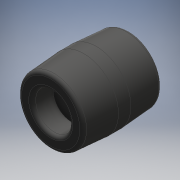
# Autodesk Inventor part: Pied
Saved by Autodesk Inventor 2016 SP1 (Build 200210100, 210)
## iProperties
Created: 2018-06-13
Part Number: Pied
Material: Caoutchouc
Document SubType Name: Modeling
Designer: dimercur
Mass: 17.4598 g
Surface Area: 52.7252 cm^2
Volume: 18.774 cm^3
Density: 0.93 g/cm^3
Appearance: Caoutchouc - Noir
Author: dimercur
Autodesk Inventor part; units mm, degrees
ref_plane "YZ Plane" through (0, 0, 0) normal (1, 0, 0) x (0, 1, 0)
ref_plane "XZ Plane" through (0, 0, 0) normal (0, 1, 0) x (-1, 0, 0)
ref_plane "XY Plane" through (0, 0, 0) normal (0, 0, 1) x (1, 0, 0)
sketch "Esquisse1" plane through (0, 0, 0) normal (0, 1, 0) x (-1, 0, 0)
  circle A0 centre (0, 0) radius 15
  dimension "d0" = 30
  constraints: 1 centre point, 1 coincident
  measures "d0" diameter of A0
extrude "Extrusion1" add sketch "Esquisse1" along normal blind 17
chamfer "Chanfrein1" distance 1 angle 86 1 edges at (15, 17, 0) measured on face at (-3.8878, 17, -2.119)
fillet "Congé1" radius 1.5 1 edges at (14, 17, 0)
sketch "Esquisse2" plane through (0, 17, 0) normal (0, 1, 0) x (1, 0, 0)
  circle A0 centre (0, 0) radius 8
  dimension "d7" = 16
  constraints: 1 centre point, 1 coincident
  measures "d7" diameter of A0
extrude "Extrusion2" cut sketch "Esquisse2" against normal blind 9
fillet "Congé2" radius 1.5 1 edges at (-8, 17, 0)
sketch "Esquisse3" plane through (0, 0, 0) normal (0, -1, 0) x (1, 0, 0)
  circle A0 centre (0, 0) radius 2
  dimension "d11" = 4
  constraints: 1 centre point, 1 coincident
  measures "d11" diameter of A0
extrude "Extrusion3" cut sketch "Esquisse3" against normal blind 9
mirror "Symétrie1" about plane through (0, 0, 0) normal (0, -1, 0) of "Extrusion1", "Chanfrein1", "Congé1", "Extrusion2", "Congé2", "Extrusion3"
